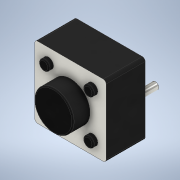
# Autodesk Inventor part: Button
Saved by Autodesk Inventor 2020 (Build 240168000, 168)
## iProperties
Created: 2021-01-14
Part Number: Button
Material: Generic
Document SubType Name: Modeling
Designer: Luke
Density: 1 g/cm^3
Appearance: Default
Author: Luke
Autodesk Inventor part; units mm, degrees
ref_plane "YZ Plane" through (0, 0, 0) normal (1, 0, 0) x (0, 1, 0)
ref_plane "XZ Plane" through (0, 0, 0) normal (0, 1, 0) x (-1, 0, 0)
ref_plane "XY Plane" through (0, 0, 0) normal (0, 0, 1) x (1, 0, 0)
ref_plane "Work Plane1" through (0, 0, 0) normal (0, 0, 1) x (1, 0, 0)
sketch "Sketch1" plane through (0, 0, 0) normal (0, 0, 1) x (1, 0, 0)
  circle A0 centre (2.54, -6.27) radius 0.302 projected
  circle A1 centre (-2.46, -6.27) radius 0.302 projected
  line L0 (2.54, -6.27) -> (-2.46, -6.27)
  line L1 (2.89, -9.37) -> (-2.81, -9.37)
  line L2 (-3.06, -9.12) -> (-3.06, -3.42)
  line L3 (-2.81, -3.17) -> (2.89, -3.17)
  line L4 (3.14, -3.42) -> (3.14, -9.12)
  line L5 (3.14, -9.37) -> (-3.06, -3.17) construction
  line L6 (-3.06, -9.37) -> (3.14, -3.17) construction
  arc A2 (2.89, -9.37) -> (3.14, -9.12) centre (2.89, -9.12) ccw
  arc A3 (-3.06, -9.12) -> (-2.81, -9.37) centre (-2.81, -9.12) ccw
  arc A4 (-2.81, -3.17) -> (-3.06, -3.42) centre (-2.81, -3.42) ccw
  arc A5 (3.14, -3.42) -> (2.89, -3.17) centre (2.89, -3.42) ccw
  point P0 (0, 0)
  point P1 (0.04, -6.27)
  dimension "d0" = 6.2
  dimension "d1" = 6.2
  dimension "d2" = 0.25
  constraints: 14 end point, 8 point on circle, 8 point on line, 8 tangent, 4 centre point, 3 equal radius, 3 midpoint, 2 horizontal, 2 parallel, 1 perpendicular
  measures "d0" distance of L5.end L6.end
  measures "d1" distance of L6.start L5.end
  measures "d2" radius of A2
extrude "Extrusion1" add sketch "Sketch1" along normal blind 3.4 contours A0 | A1 | L1 A3 L2 A4 L3 A5 L4 A2
sketch "Sketch2" plane through (0, 0, 3.4) normal (0, 0, 1) x (1, 0, 0)
  arc A0 (2.89, -9.37) -> (3.14, -9.12) centre (2.89, -9.12) ccw projected
  line L0 (3.14, -9.12) -> (3.14, -3.42) projected
  arc A1 (3.14, -3.42) -> (2.89, -3.17) centre (2.89, -3.42) ccw projected
  line L1 (2.89, -3.17) -> (-2.81, -3.17) projected
  arc A2 (-2.81, -3.17) -> (-3.06, -3.42) centre (-2.81, -3.42) ccw projected
  line L2 (-3.06, -3.42) -> (-3.06, -9.12) projected
  arc A3 (-3.06, -9.12) -> (-2.81, -9.37) centre (-2.81, -9.12) ccw projected
  line L3 (-2.81, -9.37) -> (2.89, -9.37) projected
  line L4 (-1.885, -4.345) -> (1.965, -8.195) construction
  line L5 (1.965, -4.345) -> (-1.885, -8.195) construction
  circle A4 centre (1.965, -4.345) radius 0.45
  circle A5 centre (1.965, -8.195) radius 0.45
  circle A6 centre (-1.885, -8.195) radius 0.45
  circle A7 centre (-1.885, -4.345) radius 0.45
  point P0 (0, 0)
  point P1 (0.04, -6.27)
  dimension "d5" = 3.85
  dimension "d6" = 3.85
  dimension "d7" = 0.9
  dimension "d8" = 0.9
  dimension "d9" = 0.9
  dimension "d10" = 0.9
  constraints: 4 centre point, 4 coincident, 4 end point, 2 midpoint
  measures "d5" distance of L4.end L5.end
  measures "d6" distance of L5.start L4.end
  measures "d7" diameter of A4
  measures "d8" diameter of A5
  measures "d9" diameter of A6
  measures "d10" diameter of A7
extrude "Extrusion2" add sketch "Sketch2" along normal blind 0.4 contours A4 | A5 | A6 | A7
fillet "Fillet1" radius 0.1 4 edges at (1.515, -4.345, 3.8) (1.515, -8.195, 3.8) (-2.335, -8.195, 3.8) (-2.335, -4.345, 3.8)
sketch "Sketch3" plane through (0, 0, 3.4) normal (0, 0, 1) x (1, 0, 0)
  circle A0 centre (-1.885, -8.195) radius 0.45 projected
  circle A1 centre (1.965, -8.195) radius 0.45 projected
  circle A2 centre (-1.885, -4.345) radius 0.45 projected
  circle A3 centre (1.965, -4.345) radius 0.45 projected
  arc A4 (2.89, -9.37) -> (3.14, -9.12) centre (2.89, -9.12) ccw projected
  line L0 (3.14, -9.12) -> (3.14, -3.42) projected
  arc A5 (3.14, -3.42) -> (2.89, -3.17) centre (2.89, -3.42) ccw projected
  line L1 (2.89, -3.17) -> (-2.81, -3.17) projected
  arc A6 (-2.81, -3.17) -> (-3.06, -3.42) centre (-2.81, -3.42) ccw projected
  line L2 (-3.06, -3.42) -> (-3.06, -9.12) projected
  arc A7 (-3.06, -9.12) -> (-2.81, -9.37) centre (-2.81, -9.12) ccw projected
  line L3 (-2.81, -9.37) -> (2.89, -9.37) projected
  circle A8 centre (0.04, -6.27) radius 1.7
  point P0 (0, 0)
  dimension "d14" = 3.4
  constraints: 1 centre point, 1 coincident
  measures "d14" diameter of A8
extrude "Extrusion3" add sketch "Sketch3" along normal blind 1.48 contours A8
fillet "Fillet2" radius 0.1 1 edges at (-1.66, -6.27, 4.88)
sketch "Sketch4" plane through (0, 0, 0) normal (0, 0, -1) x (-1, 0, 0)
  circle A0 centre (2.46, -6.27) radius 0.302 projected
  circle A1 centre (-2.54, -6.27) radius 0.302 projected
  point P0 (0, 0)
extrude "Extrusion4" add sketch "Sketch4" along normal blind 1.48
body "Solid1"
